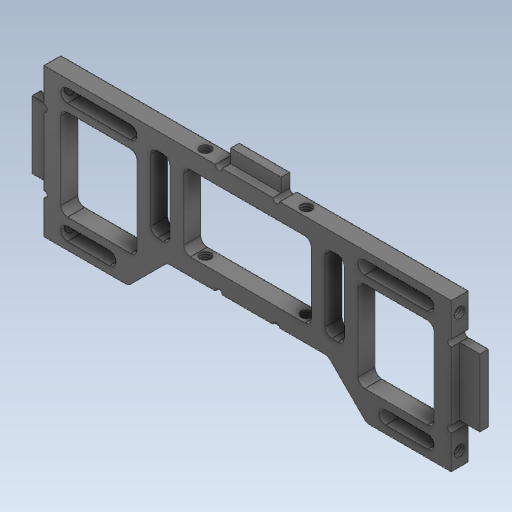
# Autodesk Inventor part: Trunk_chest_frame
Saved by Autodesk Inventor 2020.4 (Build 244396000, 396)
## iProperties
Created: 2022-01-02
Part Number: Trunk_chest_frame
Material: アセタール樹脂、黒
Document SubType Name: Modeling
Designer: Masato Kubotera
Density: 1.425 g/cm^3
Appearance: 滑らか - 黒
Mass: 14.4249 g
Surface Area: 93.8511 cm^2
Volume: 10.1227 cm^3
Description: POM T5
Author: Masato Kubotera
Autodesk Inventor part; units mm, degrees
ref_plane "YZ Plane" through (0, 0, 0) normal (1, 0, 0) x (0, 1, 0)
ref_plane "XZ Plane" through (0, 0, 0) normal (0, 1, 0) x (-1, 0, 0)
ref_plane "XY Plane" through (0, 0, 0) normal (0, 0, 1) x (1, 0, 0)
sketch "スケッチ1" plane through (0, 0, 0) normal (0, 0, 1) x (1, 0, 0)
  line L0 (-60.5, 22) -> (60.5, 22) construction
  line L1 (60.5, 22) -> (60.5, -22) construction
  line L2 (60.5, -22) -> (-60.5, -22) construction
  line L3 (-60.5, -22) -> (-60.5, 22) construction
  line L4 (-60.5, 22) -> (60.5, -22) construction
  line L5 (60.5, 22) -> (-60.5, -22) construction
  line L6 (-60.5, 0) -> (60.5, 0) construction
  line L7 (-60.5, 5.75) -> (60.5, 5.75) construction
  line L8 (0, 22) -> (0, -22) construction
  line L9 (-60.5, 0) -> (60.5, 0) construction
  line L10 (7.5, 26) -> (-7.5, 26)
  line L11 (-7.5, 26) -> (-7.5, 22)
  arc A0 (-9.6, 22) -> (-7.5, 22) centre (-8.55, 22) ccw
  line L12 (-15, 22) -> (-15, -10.5) construction
  line L13 (-60.5, -10.5) -> (60.5, -10.5) construction
  line L14 (7.5, 26) -> (7.5, 22)
  arc A1 (7.5, 22) -> (9.6, 22) centre (8.55, 22) ccw
  line L15 (15, 22) -> (15, -10.5) construction
  line L16 (-60.5, 16) -> (60.5, 16) construction
  line L17 (-23, 16) -> (-23, -16) construction
  line L18 (-34.8, 16) -> (-34.8, -16) construction
  line L19 (-60.5, -16) -> (60.5, -16) construction
  line L20 (-53.5, 13.5) -> (-34.8, 13.5)
  line L21 (-32.8, 11.5) -> (-32.8, -11.5)
  line L22 (-34.8, -13.5) -> (-53.5, -13.5)
  line L23 (-55.5, -11.5) -> (-55.5, 11.5)
  line L24 (-55.5, 13.5) -> (-32.8, -13.5) construction
  line L25 (-32.8, 13.5) -> (-55.5, -13.5) construction
  arc A2 (-53.5, 13.5) -> (-55.5, 11.5) centre (-53.5, 11.5) ccw
  arc A3 (-55.5, -11.5) -> (-53.5, -13.5) centre (-53.5, -11.5) ccw
  arc A4 (-34.8, -13.5) -> (-32.8, -11.5) centre (-34.8, -11.5) ccw
  arc A5 (-32.8, 11.5) -> (-34.8, 13.5) centre (-34.8, 11.5) ccw
  line L26 (-60.5, -22) -> (-36.2289, -22)
  line L27 (-60.5, 22) -> (-9.6, 22)
  line L28 (-53.5, 19.75) -> (-34.8, 19.75)
  line L29 (-32.8, 17.75) -> (-32.8, 17.75)
  line L30 (-34.8, 15.75) -> (-53.5, 15.75)
  line L31 (-55.5, 17.75) -> (-55.5, 17.75)
  line L32 (-55.5, 19.75) -> (-32.8, 15.75) construction
  line L33 (-32.8, 19.75) -> (-55.5, 15.75) construction
  line L34 (-23, 22) -> (-23, 26) construction
  line L35 (-23, 26) -> (23, 26) construction
  line L36 (23, 26) -> (23, 22) construction
  line L37 (23, 22) -> (-23, 26) construction
  line L38 (-23, 22) -> (23, 26) construction
  line L39 (-19, 26) -> (-19, -16) construction
  line L40 (-60.5, 10) -> (-66.5, 10)
  line L41 (-66.5, 10) -> (-66.5, -10)
  line L42 (-60.5, -10) -> (-66.5, -10)
  arc A6 (-60.5, 10) -> (-60.5, 12.1) centre (-60.5, 11.05) ccw
  arc A7 (-60.5, -12.1) -> (-60.5, -10) centre (-60.5, -11.05) ccw
  line L43 (-60.5, 22) -> (-60.5, 12.1)
  line L44 (-60.5, -12.1) -> (-60.5, -22)
  arc A8 (-53.5, 19.75) -> (-55.5, 17.75) centre (-53.5, 17.75) ccw
  arc A9 (-55.5, 17.75) -> (-53.5, 15.75) centre (-53.5, 17.75) ccw
  arc A10 (-32.8, 17.75) -> (-34.8, 19.75) centre (-34.8, 17.75) ccw
  arc A11 (-34.8, 15.75) -> (-32.8, 17.75) centre (-34.8, 17.75) ccw
  line L45 (-55.5, 17.75) -> (-60.5, 17.75) construction
  line L46 (-60.5, 15.75) -> (-56.5, 15.75) construction
  line L47 (-60.5, 19.75) -> (-56.5, 19.75) construction
  line L48 (-53.5, -19.75) -> (-41.05, -19.75)
  arc A12 (-55.5, -17.75) -> (-53.5, -19.75) centre (-53.5, -17.75) ccw
  arc A13 (-53.5, -15.75) -> (-55.5, -17.75) centre (-53.5, -17.75) ccw
  line L49 (-55.5, -17.75) -> (-60.5, -17.75) construction
  line L50 (-60.5, -15.75) -> (-56.5, -15.75) construction
  line L51 (-60.5, -19.75) -> (-56.5, -19.75) construction
  line L52 (-55.5, -17.75) -> (-55.5, -17.75)
  line L53 (0, 26) -> (0, -12.5)
  line L54 (-60.5, 10) -> (-60.5, -10)
  line L55 (-7.5, 22) -> (7.5, 22)
  line L56 (-26.8, 17) -> (-25, 17)
  line L57 (-23, 15) -> (-23, -3.5)
  line L58 (-25, -5.5) -> (-26.8, -5.5)
  line L59 (-28.8, 17) -> (-23, -5.5) construction
  line L60 (-23, 17) -> (-28.8, -5.5) construction
  arc A14 (-26.8, 17) -> (-28.8, 15) centre (-26.8, 15) ccw
  arc A15 (-23, 15) -> (-25, 17) centre (-25, 15) ccw
  arc A16 (-25, -5.5) -> (-23, -3.5) centre (-25, -3.5) ccw
  arc A17 (-28.8, -3.5) -> (-26.8, -5.5) centre (-26.8, -3.5) ccw
  line L61 (17, 17) -> (-17, 17)
  line L62 (-19, 15) -> (-19, -3.5)
  line L63 (-17, -5.5) -> (17, -5.5)
  line L64 (19, -3.5) -> (19, 15)
  line L65 (19, 17) -> (-19, -5.5) construction
  line L66 (-19, 17) -> (19, -5.5) construction
  arc A18 (-17, 17) -> (-19, 15) centre (-17, 15) ccw
  arc A19 (-19, -3.5) -> (-17, -5.5) centre (-17, -3.5) ccw
  arc A20 (17, -5.5) -> (19, -3.5) centre (17, -3.5) ccw
  arc A21 (19, 15) -> (17, 17) centre (17, 15) ccw
  line L67 (-28.8, 15) -> (-28.8, -3.5)
  line L68 (-34.8147, -21.4142) -> (-24.4863, -11.0858)
  line L69 (-39.6358, -19.1642) -> (-39.6358, -19.1642)
  line L70 (-41.05, -15.75) -> (-53.5, -15.75)
  arc A22 (-39.6358, -19.1642) -> (-41.05, -15.75) centre (-41.05, -17.75) ccw
  arc A23 (-41.05, -19.75) -> (-39.6358, -19.1642) centre (-41.05, -17.75) ccw
  line L71 (-23.0721, -10.5) -> (0, -10.5)
  arc A24 (-7.5, -10.5) -> (-9.6, -10.5) centre (-8.55, -10.5) ccw
  arc A25 (9.6, -10.5) -> (7.5, -10.5) centre (8.55, -10.5) ccw
  line L72 (-7.5, -10.5) -> (7.5, -10.5)
  arc A26 (-23.0721, -10.5) -> (-24.4863, -11.0858) centre (-23.0721, -12.5) ccw
  arc A27 (-36.2289, -22) -> (-34.8147, -21.4142) centre (-36.2289, -20) ccw
  line L73 (-7.5, -10.5) -> (-7.5, -12.5)
  line L74 (-7.5, -12.5) -> (7.5, -12.5)
  line L75 (7.5, -12.5) -> (7.5, -10.5)
  point P0 (0, 0)
  point P1 (-44.15, 0)
  point P2 (-35.4005, -22)
  point P3 (-44.15, 17.75)
  point P4 (0, 24)
  point P5 (0, 24)
  point P6 (0, 22)
  point P7 (-25.9, 5.75)
  point P8 (0, 5.75)
  point P9 (0, -5.5)
  point P10 (0, 17)
  point P11 (-23.9005, -10.5)
  point P12 (0, -10.5)
  point P13 (-9.6, -10.5)
  point P14 (-55.5, -17.75)
  point P15 (-55.5, 17.75)
  dimension "d0" = 121
  dimension "d3" = 16.25
  dimension "d4" = 1.05
  dimension "d5" = 32.5
  dimension "d6" = 30
  dimension "d7" = 15
  dimension "d8" = 4
  dimension "d12" = 11.8
  dimension "d13" = 32
  dimension "d14" = 16
  dimension "d15" = 6
  dimension "d16" = 2
  dimension "d18" = 2
  dimension "d19" = 5
  dimension "d20" = 5.5
  dimension "d21" = 6
  dimension "d26" = 27
  dimension "d29" = 4
  dimension "d31" = 4
  dimension "d32" = 1.05
  dimension "d33" = 6
  dimension "d34" = 20
  dimension "d35" = 8.5
  dimension "d36" = 4.25
  dimension "d37" = 2
  dimension "d38" = 4
  dimension "d39" = 35.5
  dimension "d67" = 44
  dimension "d81" = 2
  dimension "d87" = 2
  dimension "d88" = 5
  dimension "d90" = 4
  dimension "d91" = 4
  dimension "d98" = 4
  dimension "d99" = 5.75
  dimension "d100" = 5
  dimension "d101" = 45
  dimension "d102" = 2
  dimension "d103" = 38
  dimension "d112" = 2
  dimension "d120" = 2
  constraints: 150 end point, 60 point on line, 56 point on circle, 41 tangent, 30 symmetric about line, 28 centre point, 22 midpoint, 17 perpendicular, 14 equal radius, 12 parallel, 11 horizontal, 9 collinear, 5 vertical, 18 other
  measures "d0" distance of L1.end L2.end
  measures "d3" distance of L7.start L0.start
  measures "d4" radius of A0
  measures "d5" distance of L13.start L0.start
  measures "d6" distance of L15.start L12.start
  measures "d7" distance of L10.start L10.end
  measures "d8" distance of L10.start L14.end
  measures "d12" distance of L17.start L18.start
  measures "d13" distance of L16.start L19.start
  measures "d14" distance of L19.start L6.start
  measures "d15" distance of L2.end L19.start
  measures "d16" radius of A2
  measures "d18" distance between parallel lines of L21 L18
  measures "d19" distance from line of L0.start L23
  measures "d20" distance of L19.start L13.start
  measures "d21" distance of L16.start L0.start
  measures "d26" distance of L22.start L20.end
  measures "d29" distance of L33.start L32.end
  measures "d31" distance of L34.end L39.start
  measures "d32" radius of A6
  measures "d33" distance of L40.end L40.start
  measures "d34" distance of L40.end L41.end
  measures "d35" vertical distance of L20.start L0.start
  measures "d36" vertical distance of L0.start point (-44.15, 17.75)
  measures "d37" radius of A8
  measures "d38" distance of L46.end L47.end
  measures "d39" distance of L49.end L45.end
  measures "d67" distance of L2.end L0.start
  measures "d81" radius of A14
  measures "d87" radius of A18
  measures "d88" distance between parallel lines of L61 L0
  measures "d90" distance between parallel lines of L21 L67
  measures "d91" distance between parallel lines of L62 L57
  measures "d98" horizontal distance of L34.start L62.start
  measures "d99" distance of L6.start L7.start
  measures "d100" distance between parallel lines of L69 L68
  measures "d101" angle of L68 L26
  measures "d102" radius of A22
  measures "d103" distance between parallel lines of L64 L62
  measures "d112" radius of A26
  measures "d120" distance of L73.end L72.start
extrude "押し出し1" add sketch "スケッチ1" along normal blind 5 contours L53 L61 A18 L62 A19 L63 L71 A24 A26 L68 A27 L26 L44 A7 L54 A6 L43 L27 A0 L55
extrude "押し出し2" add sketch "スケッチ1" along normal blind 2.5 contours L53 L55 L11 L10 | L53 L74 L73 L71 | L54 L42 L41 L40
sketch "スケッチ2" plane through (-60.5, 12.1, 0) normal (-1, 0, 0) x (0, 0, 1)
  line L0 (2.5, 9.9) -> (2.5, -34.1)
  line L1 (0, -34.1) -> (5, -34.1) projected
  line L2 (0, -12.1) -> (5, -12.1)
  line L3 (0, 9.9) -> (5, 9.9) projected
  line L4 (5, -2.1) -> (5, -22.1) projected
  point P0 (2.5, 5.65)
  point P1 (2.5, -29.85)
  dimension "d42" = 35.5
  constraints: 4 end point, 3 midpoint, 2 point on line, 1 symmetric about line
  measures "d42" distance of point (2.5, -29.85) point (2.5, 5.65)
hole "穴1" at (-60.5, -17.75, 2.5) at (-60.5, 17.75, 2.5) direction (1, 0, 0) diameter 3.242 depth 6 tip angle 118 thread size "M4x0.7" class "6H" standard "ISO Metric profile"
sketch "スケッチ3" plane through (-60.5, 22, 0) normal (0, 1, 0) x (1, 0, 0)
  line L0 (0, 0) -> (0, -5) projected
  line L1 (0, -2.5) -> (60.5, -2.5)
  line L2 (0, 0) -> (0, -5) projected
  line L3 (60.5, 0) -> (60.5, -2.5) projected
  point P0 (45.5, -2.5)
  dimension "d104" = 15
  constraints: 2 end point, 2 midpoint, 1 horizontal, 1 point on line
  measures "d104" distance from line of point (45.5, -2.5) L3
hole "穴2" at (-15, 22, 2.5) direction (0, -1, 0) diameter 3.242 depth 5 tip angle 118 thread size "M4x0.7" class "6H" standard "ISO Metric profile"
sketch "スケッチ4" plane through (-23.0721, -10.5, 5) normal (0, -1, 0) x (1, 0, 0)
  circle A0 centre (8.0721, -2.5) radius 1.621 projected
  point P0 (23.0721, -5)
  constraints: 1 coincident
hole "穴3" at (-15, -10.5, 2.5) direction (0, 1, 0) diameter 3.242 depth 5 tip angle 118 thread size "M4x0.7" class "6H" standard "ISO Metric profile"
mirror "ミラー1" about plane through (0, -10.5, 0) normal (1, 0, 0)
equation "\"d3\" = 0.5 * d5"
equation "\"d14\" = 0.5 * d13"
equation "\"d32\" = d4"
